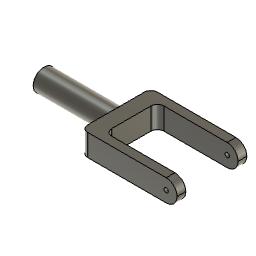
wheel_holder (Autodesk Fusion 360 design; units mm, degrees)
Autodesk Fusion 360 part; units mm, degrees
ref_plane "WorkPlane1" through (4, 0, 0) normal (1, 0, 0) x (0, 1, 0)
sketch "Sketch2" plane through (0, 0, 0) normal (1, 0, 0) x (0, 1, 0)
  line L0 (-12, 0) -> (-16, 0)
  line L1 (-16, 0) -> (-16, 5)
  line L2 (-16, 5) -> (-12, 5)
  line L3 (-12, 5) -> (-12, 0)
  line L4 (12, 0) -> (16, 0)
  line L5 (16, 0) -> (16, 5)
  line L6 (16, 5) -> (12, 5)
  line L7 (12, 5) -> (12, 0)
  line L8 (-12, 5) -> (12, 5)
  line L9 (12, 5) -> (12, 0)
  line L10 (12, 0) -> (-12, 0)
  line L11 (-12, 0) -> (-12, 5)
  constraint horizontal L0
  constraint vertical L1
  constraint horizontal L2
  constraint vertical L3
  constraint horizontal L4
  constraint vertical L5
  constraint horizontal L6
  constraint vertical L7
  constraint horizontal L8
  constraint vertical L9
  constraint horizontal L10
  constraint vertical L11
extrude "Extrude1" add sketch "Sketch2" along normal blind 7 contours L3 L7 L8 L9 L10 L11 makes body 1
extrude "Extrude2" add sketch "Sketch2" along normal blind 44 separate body contours L0 L1 L2 L3 L11 | L4 L5 L6 L7 L9 makes body 2 at (29.3333, -16, 1.6667) makes body 3 at (29.3333, 12, 3.3333)
fillet "Fillet1" radius 5 2 edges at (44, -14, 5) (44, 14, 5) on bodies 2 3
sketch "Sketch3" plane through (0, 0, 0) normal (0, 1, 0) x (1, 0, 0)
  circle A0 centre (39, 0) radius 1
  dimension "d8" = 2
  measures "d8" diameter of A0
sketch "Sketch4" plane through (0, 0, 0) normal (1, 0, 0) x (0, 1, 0)
  circle A0 centre (0, 0) radius 5
  constraint coincident A0.centre origin
extrude "Extrude4" add sketch "Sketch4" against normal blind 33 bodies 1
shell "Shell1" thickness 2 removed faces 1 at (-33, -1.5016, -0.7231) on bodies 1
ref_plane "WorkPlane2" through (-2, 0, 0) normal (1, 0, 0) x (0, 1, 0)
sketch "Sketch7" plane through (-2, 0, 0) normal (1, 0, 0) x (0, 1, 0)
sketch "Sketch8" plane through (0, 0, 0) normal (1, 0, 0) x (0, 1, 0)
  circle A0 centre (0, 0) radius 3
  constraint coincident A0.centre origin
extrude "Extrude6" add sketch "Sketch8" against normal blind 29 bodies 1
extrude "Extrude8" add 5 faces at (2.3333, 9.6667, 0) (14.6667, -13.3333, 0) (14.6667, 13.3333, 0) (14.6667, 13.3333, 0) (14.6667, -13.3333, 0) along direction (0, 0, -1) blind 5 on bodies 1 2 3 bodies 1 2 3
fillet "Fillet2" radius 5 2 edges at (44, 14, -5) (44, -14, -5) on bodies 1
extrude "Extrude12" cut sketch "Sketch3" along normal mid plane 48 bodies 1
fillet "Fillet3" radius 3 2 edges at (0, -16, 0) (0, 16, 0) on bodies 1
fillet "Fillet4" radius 3 2 edges at (7, -12, 0) (7, 12, 0) on bodies 1
